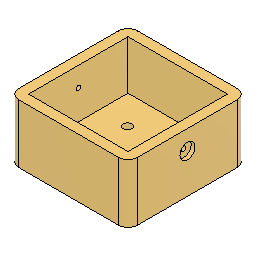
Caster Adapter to Leg v5 (Autodesk Fusion 360 design; units mm, degrees)
Autodesk Fusion 360 part; units mm, degrees
note: some values were not read from the file. Chosen so that the rebuilt part matches the saved one: which face or edge a step refers to.
box "BoxPrimitive1" add length 60.8 width 60.8 height 30 placed x (0, 0, 1) y (1, 0, 0) z (0, 1, 0) at (0, 0, 0) makes body 1
sketch "Sketch2" plane through (0, 30, 0) normal (0, 1, 0) x (-1, 0, 0)
  line L0 (0, 60.8) -> (-60.8, 60.8)
  line L1 (-60.8, 60.8) -> (-60.8, 0)
  line L2 (-60.8, 0) -> (0, 0)
  line L3 (0, 0) -> (0, 60.8)
  line L4 (0, 0) -> (-5, 0)
  line L5 (-5, 0) -> (-5, 5)
  line L6 (-5, 5) -> (-5, 55.8)
  line L7 (-5, 55.8) -> (-55.8, 55.8)
  line L8 (-55.8, 55.8) -> (-55.8, 5)
  line L9 (-55.8, 5) -> (-5, 5)
extrude "Extrude1" cut sketch "Sketch2" against normal blind 25 contours L6 L7 L8 L9 bodies 1
fillet "Fillet1" radius 5 4 edges at (60.8, 15, 0) (0, 15, 0) (0, 15, 60.8) (60.8, 15, 60.8) on bodies 1
sketch "Sketch3" plane through (0, 0, 0) normal (0, -1, 0) x (1, 0, 0)
  arc A0 (60.8, 55.8) -> (55.8, 60.8) centre (55.8, 55.8) ccw
  line L0 (55.8, 60.8) -> (5, 60.8)
  arc A1 (5, 60.8) -> (0, 55.8) centre (5, 55.8) ccw
  line L1 (0, 55.8) -> (0, 5)
  arc A2 (0, 5) -> (5, 0) centre (5, 5) ccw
  line L2 (5, 0) -> (55.8, 0)
  arc A3 (55.8, 0) -> (60.8, 5) centre (55.8, 5) ccw
  line L3 (60.8, 5) -> (60.8, 55.8)
  line L4 (0, 0) -> (0, 60.8)
  line L5 (0, 60.8) -> (60.8, 60.8)
  line L6 (60.8, 60.8) -> (60.8, 0)
  line L7 (60.8, 0) -> (55.8, 0)
  line L8 (60.8, 0) -> (60.8, 15.3)
  line L9 (60.8, 60.8) -> (60.8, 45.5)
  line L10 (60.8, 15.3) -> (45.5, 15.3)
  line L11 (45.5, 15.3) -> (45.5, 45.5)
  line L12 (45.5, 45.5) -> (15.3, 45.5)
  line L13 (15.3, 45.5) -> (15.3, 15.3)
  line L14 (15.3, 15.3) -> (45.5, 15.3)
  line L15 (45.5, 15.3) -> (45.5, 17.3)
  line L16 (45.5, 17.3) -> (43.5, 17.3)
  line L17 (43.5, 17.3) -> (43.5, 19.8)
  line L18 (43.5, 19.8) -> (41, 19.8)
  circle A4 centre (41, 19.8) radius 2.2
  line L19 (45.5, 45.5) -> (45.5, 43.5)
  line L20 (45.5, 43.5) -> (43.5, 43.5)
  line L21 (43.5, 43.5) -> (43.5, 41)
  line L22 (43.5, 41) -> (41, 41)
  circle A5 centre (41, 41) radius 2.2
  line L23 (41, 41) -> (19.5, 41) construction
  line L24 (19.5, 41) -> (19.5, 19.8) construction
  line L25 (19.5, 19.8) -> (41, 19.8) construction
  circle A6 centre (19.5, 41) radius 2.2
  circle A7 centre (19.5, 19.8) radius 2.2
  dimension "d9" = 15.3
  dimension "d10" = 15.3
extrude "Extrude2" cut sketch "Sketch3" against normal blind 9 contours A4 | A5 | A6 | A7 bodies 1
sketch "Sketch4" plane through (60.8, 0, 0) normal (1, 0, 0) x (0, 0, -1)
  line L0 (-55.8, 30) -> (-55.8, 0)
  line L1 (-55.8, 0) -> (-5, 0)
  line L2 (-5, 0) -> (-5, 30)
  line L3 (-5, 30) -> (-55.8, 30)
  line L4 (-55.8, 30) -> (-55.8, 20) construction
  line L5 (-55.8, 20) -> (-5, 20) construction
  line L6 (-30.4, 20) -> (-30.4, 30) construction
  circle A0 centre (-30.4, 20) radius 1.15
  circle A1 centre (-30.4, 20) radius 3.875
extrude "Extrude3" cut sketch "Sketch4" against normal blind 2 contours A1 bodies 1
extrude "Extrude4" cut 1 faces at (60.8, 19.6263, 30.4853) along direction (-1, 0, 0) blind 56.5 on bodies 1 bodies 1
extrude "Extrude5" cut 1 faces at (4.3, 19.6263, 30.4853) along direction (-1, 0, 0) blind 45 on bodies 1 bodies 1
cylinder "CylinderPrimitive1" cut diameter 7.75 height -2 placed x (0, 0, 1) y (0, 1, 0) z (-1, 0, 0) at (0, 20, 30.4) bodies 1
copy_body "Body->Comp1" bodies 1 removing the originals makes body 2 in component "Caster to IKEA Lack Leg Adapter"
component "Caster to IKEA Lack Leg Adapter" placed x (1, 0, 0) y (0, 1, 0) z (0, 0, 1) at (0, 0, 0)
equation "d9 = ( 60.800 mm - 30.2 mm ) / 2"
